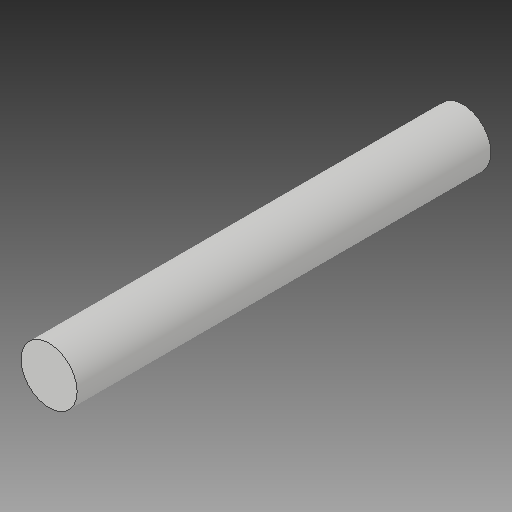
# Autodesk Inventor part: 5mmRod
Saved by Autodesk Inventor 2019 (Build 230136000, 136)
## iProperties
Created: 2019-05-16
Part Number: 5mmRod
Material: Generic
Document SubType Name: Modeling
Designer: Alex Jones
Density: 1 g/cm^3
Appearance: Default
Author: Alex Jones
Autodesk Inventor part; units mm, degrees
ref_plane "YZ Plane" through (0, 0, 0) normal (1, 0, 0) x (0, 1, 0)
ref_plane "XZ Plane" through (0, 0, 0) normal (0, 1, 0) x (-1, 0, 0)
ref_plane "XY Plane" through (0, 0, 0) normal (0, 0, 1) x (1, 0, 0)
sketch "Sketch1" plane through (0, 0, 0) normal (0, 0, 1) x (1, 0, 0)
  circle A0 centre (-42.4, 22.4116) radius 2.5 projected
  circle A1 centre (42.4, 22.4116) radius 2.5 projected
  circle A2 centre (20, -27.6384) radius 2.5 projected
  circle A3 centre (20, 15.1616) radius 2.5 projected
  circle A4 centre (-20, -27.6384) radius 2.5 projected
  circle A5 centre (-20, 15.1616) radius 2.5 projected
  line L0 (-26.765, 25.1616) -> (26.765, 25.1616) projected
  line L1 (-54.9, 5.1616) -> (-54.9, 12.6256) projected
  line L2 (-29.9, -19.8384) -> (-54.9, 5.1616) projected
  line L3 (-29.9, -37.5384) -> (-29.9, -19.8384) projected
  line L4 (29.9, -37.5384) -> (-29.9, -37.5384) projected
  line L5 (29.9, -19.8384) -> (29.9, -37.5384) projected
  line L6 (54.9, 5.1616) -> (29.9, -19.8384) projected
  line L7 (54.9, 12.6256) -> (54.9, 5.1616) projected
  circle A6 centre (510.0548, 24.9116) radius 2.5 projected
  circle A7 centre (510.0548, 24.9116) radius 4.7
  line L8 (510.0548, 29.6116) -> (-194.5766, 29.6116)
  line L9 (510.0548, 20.2116) -> (-194.5766, 20.2116)
  arc A8 (54.9, 12.6256) -> (26.765, 25.1616) centre (42.4, 22.4116) ccw projected
  arc A9 (-26.765, 25.1616) -> (-54.9, 12.6256) centre (-42.4, 22.4116) ccw projected
  point P0 (0, 0)
  dimension "d0" = 9.4
  constraints: 4 end point, 2 horizontal, 2 point on circle, 2 tangent, 1 centre point, 1 coincident
  measures "d0" diameter of A7
ref_plane "Work Plane1" through (-54.9, -37.5384, -36.9) normal (0, 0, -1) x (0, 1, 0)
extrude "Extrusion1" add sketch "Sketch1" against normal up to surface (36.9 mm away) contours L9 A1 | A1 L9
body "Solid1"
